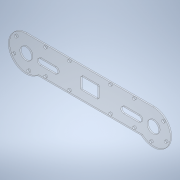
# Autodesk Inventor part: Mech Panel v7 skin exterior
Saved by Autodesk Inventor 2022 (Build 260153000, 153)
## iProperties
Created: 2022-09-24
Part Number: Mech Panel v7 skin exterior
Material: Polycarbonate, Clear
Document SubType Name: Modeling
Designer: matt
Density: 1.2 g/cm^3
Appearance: Polycarbonate - Clear
Mass: 68.4791 g
Surface Area: 427.605 cm^2
Volume: 57.0659 cm^3
Author: matt
Autodesk Inventor part; units mm, degrees
ref_plane "YZ Plane" through (0, 0, 0) normal (1, 0, 0) x (0, 1, 0)
ref_plane "XZ Plane" through (0, 0, 0) normal (0, 1, 0) x (-1, 0, 0)
ref_plane "XY Plane" through (0, 0, 0) normal (0, 0, 1) x (1, 0, 0)
sketch "Sketch3" plane through (0, 0, 0) normal (0, 0, 1) x (1, 0, 0)
  circle A0 centre (46.0375, -6) radius 3.35
  circle A1 centre (46.0375, -67.15) radius 3.35
  circle A2 centre (5.6371, -75.5294) radius 3.35
  circle A3 centre (-30.1464, -57.7223) radius 3.35
  circle A4 centre (-24.2686, -18.1875) radius 3.35
  line L0 (152.6937, 0) -> (152.6937, -73.15) construction
  line L1 (0, 0) -> (152.6937, 0)
  arc A5 (0, 0) -> (28.1723, -73.15) centre (0, -42) ccw
  line L2 (152.6937, -73.15) -> (28.1723, -73.15)
  arc A6 (24.0029, -27.5826) -> (10.7567, -16.1486) centre (0, -42) ccw
  circle A7 centre (0, -42) radius 14.224
  line L3 (9.525, -14) -> (9.525, -14.3021)
  arc A8 (11.525, -12) -> (9.525, -14) centre (11.525, -14) ccw
  arc A9 (9.525, -14.3021) -> (10.7567, -16.1486) centre (11.525, -14.3021) ccw
  arc A10 (24.0029, -27.5826) -> (25.7174, -28.5528) centre (25.7174, -26.5528) ccw
  line L4 (152.6937, -73.15) -> (277.2151, -73.15)
  line L5 (305.3873, 0) -> (152.6937, 0)
  circle A11 centre (259.3498, -6) radius 3.35
  circle A12 centre (259.3498, -67.15) radius 3.35
  circle A13 centre (299.7503, -75.5294) radius 3.35
  circle A14 centre (335.5338, -57.7223) radius 3.35
  circle A15 centre (329.6559, -18.1875) radius 3.35
  arc A16 (277.2151, -73.15) -> (305.3873, 0) centre (305.3873, -42) ccw
  arc A17 (294.6307, -16.1486) -> (281.3845, -27.5826) centre (305.3873, -42) ccw
  circle A18 centre (305.3873, -42) radius 14.224
  line L6 (295.8623, -14) -> (295.8623, -14.3021)
  arc A19 (295.8623, -14) -> (293.8623, -12) centre (293.8623, -14) ccw
  arc A20 (294.6307, -16.1486) -> (295.8623, -14.3021) centre (293.8623, -14.3021) ccw
  arc A21 (279.67, -28.5528) -> (281.3845, -27.5826) centre (279.67, -26.5528) ccw
  line L7 (34.2736, -42.1004) -> (70.2455, -42.1004) construction
  line L8 (34.2736, -49.1004) -> (70.2455, -49.1004)
  line L9 (70.2455, -35.1004) -> (34.2736, -35.1004)
  arc A22 (34.2736, -35.1004) -> (34.2736, -49.1004) centre (34.2736, -42.1004) ccw
  arc A23 (70.2455, -49.1004) -> (70.2455, -35.1004) centre (70.2455, -42.1004) ccw
  line L10 (271.1137, -42.1004) -> (235.1419, -42.1004) construction
  line L11 (271.1137, -49.1004) -> (235.1419, -49.1004)
  line L12 (235.1419, -35.1004) -> (271.1137, -35.1004)
  arc A24 (271.1137, -49.1004) -> (271.1137, -35.1004) centre (271.1137, -42.1004) ccw
  arc A25 (235.1419, -35.1004) -> (235.1419, -49.1004) centre (235.1419, -42.1004) ccw
  circle A26 centre (103.364, -67.15) radius 3.35 projected
  circle A27 centre (202.0233, -67.15) radius 3.35 projected
  circle A28 centre (202.0233, -6) radius 3.35
  circle A29 centre (103.364, -6) radius 3.35
  line L13 (123.1183, -11.9896) -> (152.6937, -11.9896)
  line L14 (152.6937, -11.9896) -> (152.6937, -48.232) construction
  line L15 (152.6937, -48.232) -> (123.1183, -48.232)
  line L16 (121.1183, -46.232) -> (121.1183, -13.9896)
  arc A30 (123.1183, -11.9896) -> (121.1183, -13.9896) centre (123.1183, -13.9896) ccw
  arc A31 (121.1183, -46.232) -> (123.1183, -48.232) centre (123.1183, -46.232) ccw
  line L17 (182.269, -11.9896) -> (152.6937, -11.9896)
  line L18 (152.6937, -48.232) -> (182.269, -48.232)
  line L19 (184.269, -46.232) -> (184.269, -13.9896)
  arc A32 (184.269, -13.9896) -> (182.269, -11.9896) centre (182.269, -13.9896) ccw
  arc A33 (182.269, -48.232) -> (184.269, -46.232) centre (182.269, -46.232) ccw
  point P0 (24.5596, -28.5528)
  point P1 (9.525, -15.6699)
  point P2 (280.8278, -28.5528)
  point P3 (295.8623, -15.6699)
  point P4 (52.2596, -42.1004)
  point P5 (253.1278, -42.1004)
  dimension "d38" = 28.448
  dimension "d39" = 2
  dimension "d40" = 2
  dimension "d43" = 14
  dimension "d44" = 2
  dimension "d45" = 6
  dimension "d46" = 213.3123
  constraints: 44 end point, 40 point on circle, 36 symmetric about line, 32 centre point, 12 tangent, 4 equal radius, 3 parallel, 3 point on line, 2 coincident, 2 horizontal, 1 midpoint, 1 perpendicular, 15 other
  measures "d38" diameter of A7
  measures "d39" radius of A8
  measures "d40" radius of A10
  measures "d43" diameter of A23
  measures "d44" radius of A30
  measures "d45" distance from line of L2 A1.centre
  measures "d46" distance of A12.centre A1.centre
extrude "Extrusion2" add sketch "Sketch3" along normal blind 3.175
body "Solid2"
